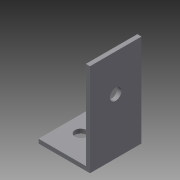
# Autodesk Inventor part: 090001-1
Saved by Autodesk Inventor 2015 (Build 190159000, 159)
## iProperties
Created: 2015-05-09
Part Number: 090001-1
Material: Generic
Document SubType Name: Modeling
Designer: Wesley
Density: 1 g/cm^3
Appearance: Default
Author: Wesley
Autodesk Inventor part; units mm, degrees
ref_plane "YZ Plane" through (0, 0, 0) normal (1, 0, 0) x (0, 1, 0)
ref_plane "XZ Plane" through (0, 0, 0) normal (0, 1, 0) x (-1, 0, 0)
ref_plane "XY Plane" through (0, 0, 0) normal (0, 0, 1) x (1, 0, 0)
sketch "Sketch1" plane through (0, 0, 0) normal (0, 1, 0) x (-1, 0, 0)
  line L0 (0, 0) -> (31.75, 0)
  line L1 (31.75, 0) -> (31.75, -31.75)
  line L2 (31.75, -31.75) -> (0, -31.75)
  line L3 (0, -31.75) -> (0, 0)
  dimension "d0" = 31.75
  dimension "d1" = 31.75
  constraints: 8 end point, 2 parallel, 1 horizontal, 1 perpendicular
  measures "d0" distance of L0.start L0.end
  measures "d1" distance of L2.end L0.start
extrude "Extrusion1" add sketch "Sketch1" along normal blind 2.54
sketch "Sketch2" plane through (0, 2.54, 0) normal (0, 1, 0) x (1, 0, 0)
  line L0 (0, 31.75) -> (-31.75, 31.75) projected
  line L1 (0, 0) -> (-2.54, 0)
  line L2 (-2.54, 0) -> (-2.54, 31.75)
  line L3 (-2.54, 31.75) -> (0, 31.75)
  line L4 (0, 31.75) -> (0, 0)
  dimension "d4" = 2.54
  constraints: 8 end point, 2 parallel, 1 horizontal, 1 perpendicular, 1 point on line
  measures "d4" distance of L2.end L3.end
extrude "Extrusion2" add sketch "Sketch2" along normal blind 54.61
sketch "Sketch3" plane through (0, 2.54, 0) normal (0, 1, 0) x (1, 0, 0)
  line L0 (-2.54, 0) -> (-2.54, 31.75) projected
  line L1 (-2.54, 31.75) -> (-31.75, 31.75) projected
  line L2 (-31.75, 31.75) -> (-31.75, 0) projected
  line L3 (-31.75, 0) -> (-2.54, 0) projected
  point P0 (0, 0)
  point P1 (-21.59, 15.875)
  dimension "d7" = 15.875
  dimension "d8" = 19.05
  measures "d7" distance from line of L3 point (-21.59, 15.875)
  measures "d8" distance from line of L0 point (-21.59, 15.875)
hole "Hole1" at (-21.59, 2.54, -15.875) direction (0, -1, 0) diameter 7.112 end through all
sketch "Sketch4" plane through (-2.54, 2.54, -31.75) normal (-1, 0, 0) x (0, 0, 1)
  line L0 (31.75, 0) -> (0, 0) projected
  line L1 (31.75, 0) -> (31.75, 54.61) projected
  line L2 (0, 54.61) -> (31.75, 54.61) projected
  line L3 (0, 0) -> (0, 54.61) projected
  point P0 (31.75, -2.54)
  point P1 (15.875, 31.75)
  dimension "d16" = 15.875
  dimension "d17" = 31.75
  measures "d16" distance from line of L3 point (15.875, 31.75)
  measures "d17" distance from line of L0 point (15.875, 31.75)
hole "Hole2" at (-2.54, 34.29, -15.875) direction (1, 0, 0) diameter 7.112 end through all
body "Solid1"
